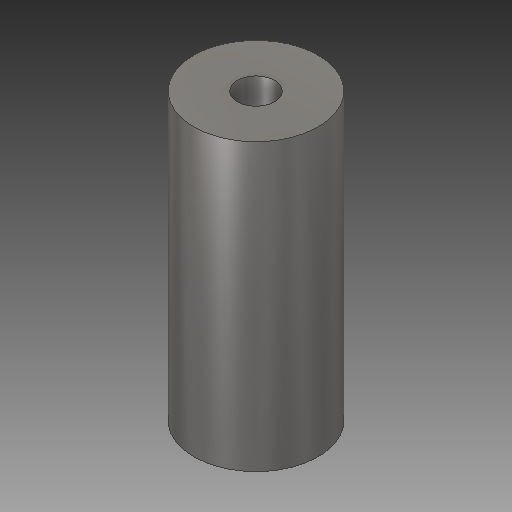
# Autodesk Inventor part: Pneumatics Connector
Saved by Autodesk Inventor 2019 (Build 230136000, 136)
## iProperties
Created: 2019-11-02
Part Number: Pneumatics Connector
Material: Stainless Steel
Document SubType Name: Modeling
Designer: admin
Density: 8 g/cm^3
Appearance: Semi-Polished
Mass: 111.087 g
Surface Area: 38.9557 cm^2
Volume: 13.8858 cm^3
Author: admin
Autodesk Inventor part; units mm, degrees
ref_plane "YZ Plane" through (0, 0, 0) normal (1, 0, 0) x (0, 1, 0)
ref_plane "XZ Plane" through (0, 0, 0) normal (0, 1, 0) x (-1, 0, 0)
ref_plane "XY Plane" through (0, 0, 0) normal (0, 0, 1) x (1, 0, 0)
sketch "Sketch1" plane through (0, 0, 0) normal (0, 1, 0) x (-1, 0, 0)
  circle A0 centre (0, 0) radius 10
  dimension "d0" = 20
  constraints: 1 centre point, 1 coincident
  measures "d0" diameter of A0
extrude "Extrusion1" add sketch "Sketch1" along normal mid plane 46
sketch "Sketch2" plane through (0, 23, 0) normal (0, 1, 0) x (1, 0, 0)
  circle A0 centre (0, 0) radius 10 projected
  constraints: 1 coincident
hole "Hole1" at (0, 23, 0) direction (0, -1, 0) diameter 6 depth 10
sketch "Sketch3" plane through (0, -23, 0) normal (0, -1, 0) x (1, 0, 0)
  circle A0 centre (0, 0) radius 10 projected
  constraints: 1 coincident
hole "Hole2" at (0, -23, 0) direction (0, 1, 0) diameter 6 depth 10
body "Solid1"
